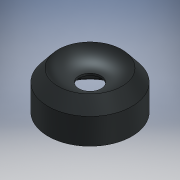
# Autodesk Inventor part: 上
Saved by Autodesk Inventor 2017 (Build 210142000, 142)
## iProperties
Part Number: 上
Material: SS41
Document SubType Name: Modeling
Designer: G
Density: 7.85 g/cm^3
Appearance: 鐵灰色
Author: G
Autodesk Inventor part; units mm, degrees
ref_plane "XZ Plane" through (0, 0, 0) normal (0, 1, 0) x (-1, 0, 0)
ref_plane "XY Plane" through (0, 0, 0) normal (0, 0, 1) x (1, 0, 0)
sketch "草圖2" plane through (11.879, 11.879, 0) normal (0, 0, -1) x (-1, 0, 0)
  circle A0 centre (-28.6785, 28.6785) radius 40.5575 projected
  point P0 (11.879, -11.879)
ref_plane "工作平面1" through (40.5575, 40.5575, 0) normal (1, 0, 0) x (0, 1, 0)
sketch "草圖3" plane through (40.5575, 40.5575, 0) normal (1, 0, 0) x (0, 1, 0)
  line L0 (-81.0575, 0) -> (-81.0575, 25)
  line L1 (-51.3075, 25) -> (-51.3075, 23)
  line L2 (-51.3075, 23) -> (-79.4575, 23)
  line L3 (-79.4575, 23) -> (-79.4575, 5)
  line L4 (-79.4575, 5) -> (-78.0575, 5)
  line L5 (-78.0575, 5) -> (-78.0575, 2)
  line L6 (-78.0575, 2) -> (-79.4575, 2)
  line L7 (-79.4575, 2) -> (-79.4575, 0)
  line L8 (-79.4575, 0) -> (-81.0575, 0)
  line L9 (-40.5575, 26.2986) -> (-40.5575, 44.6693) construction
  arc A0 (-71.3575, 37) -> (-51.3075, 25) centre (-52.0637, 46.4867) ccw
  line L10 (-81.0575, 25) -> (-71.3575, 37)
  point P0 (-40.5575, 0)
  dimension "d0" = 21.5
  dimension "d1" = 1.6
  dimension "d2" = 81
  dimension "d3" = 25
  dimension "d4" = 2
  dimension "d5" = 3
  dimension "d6" = 3
  dimension "d7" = 2
  dimension "d8" = 12
  dimension "d9" = 9.7
  dimension "d10" = 23
  dimension "d11" = 21.5
  constraints: 22 end point, 5 perpendicular, 4 point on line, 2 point on circle, 2 vertical, 1 centre point
  measures "d0" diameter of L1 L9
  measures "d1" distance between parallel lines of L0 L3
  measures "d2" diameter of L0 L9
  measures "d3" distance of L0.start L0.end
  measures "d4" distance of L1.start L1.end
  measures "d5" distance between parallel lines of L5 L0
  measures "d6" distance of L4.end L5.end
  measures "d7" distance between parallel lines of L8 L6
  measures "d8" vertical distance of L10.end L0.end
  measures "d9" horizontal distance of L10.end L0.end
  measures "d10" distance between parallel lines of L8 L2
  measures "d11" radius of A0
revolve "迴轉1" add sketch "草圖3" angle 360 about axis through (40.5575, 0, 26.2986) along (0, 0, 1)
